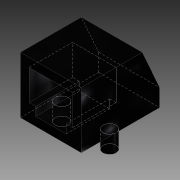
# Autodesk Inventor part: 6P6C
Saved by Autodesk Inventor 2014 (Build 180170000, 170)
## iProperties
Created: 2014-04-06
Part Number: 6P6C
Material: PC/ABS Plastic
Document SubType Name: Modeling
Designer: Tyler
Density: 0.357273 g/cm^3
Appearance: Smooth - White
Author: Tyler
Autodesk Inventor part; units mm, degrees
ref_plane "YZ Plane" through (0, 0, 0) normal (1, 0, 0) x (0, 1, 0)
ref_plane "XZ Plane" through (0, 0, 0) normal (0, 1, 0) x (-1, 0, 0)
ref_plane "XY Plane" through (0, 0, 0) normal (0, 0, 1) x (1, 0, 0)
sketch "Sketch1" plane through (0, 0, 0) normal (1, 0, 0) x (0, 1, 0)
  line L0 (-9, 13) -> (-9, 0)
  line L1 (-9, 0) -> (9, 0)
  line L2 (9, 0) -> (9, 4)
  line L3 (9, 4) -> (5, 13)
  line L4 (5, 13) -> (-9, 13)
  point P0 (0, 0)
  dimension "d0" = 13
  dimension "d1" = 18
  dimension "d2" = 9
  dimension "d3" = 0
  dimension "d4" = 4
  dimension "d5" = 14
  constraints: 10 end point, 2 parallel, 1 perpendicular, 1 vertical
  measures "d0" distance of L0.start L0.end
  measures "d1" distance of L0.end L1.end
  measures "d2" distance from line of point (0, 0) L0
  measures "d3" distance from line of L1 point (0, 0)
  measures "d4" distance of L1.end L2.end
  measures "d5" distance of L3.end L0.start
extrude "Extrusion1" add sketch "Sketch1" along normal blind 14
sketch "Sketch2" plane through (0, -9, 0) normal (0, -1, 0) x (1, 0, 0)
  line L0 (0, 13) -> (0, 0) projected
  line L1 (14, 13) -> (14, 0) projected
  line L2 (0, 13) -> (14, 13) projected
  line L3 (2, 11) -> (12, 11)
  line L4 (12, 11) -> (12, 4)
  line L5 (12, 4) -> (2, 4)
  line L6 (2, 4) -> (2, 11)
  line L7 (3.5, 2) -> (10.5, 2)
  line L8 (10.5, 2) -> (10.5, 4)
  line L9 (10.5, 4) -> (3.5, 4)
  line L10 (3.5, 4) -> (3.5, 2)
  dimension "d8" = 10
  dimension "d9" = 7
  dimension "d10" = 2
  dimension "d11" = 2
  dimension "d12" = 2
  dimension "d13" = 7
  dimension "d14" = 2
  dimension "d15" = 0
  dimension "d16" = 3.5
  constraints: 16 end point, 4 parallel, 2 horizontal, 2 perpendicular
  measures "d8" distance between parallel lines of L4 L6
  measures "d9" distance between parallel lines of L5 L3
  measures "d10" distance between parallel lines of L2 L3
  measures "d11" distance between parallel lines of L4 L1
  measures "d12" distance between parallel lines of L0 L6
  measures "d13" distance of L8.end L9.end
  measures "d14" distance of L9.end L7.start
  measures "d15" distance between parallel lines of L5 L9
  measures "d16" distance between parallel lines of L0 L10
extrude "Extrusion2" cut sketch "Sketch2" against normal blind 10
sketch "Sketch3" plane through (0, -9, 0) normal (0, 0, -1) x (-1, 0, 0)
  line L0 (0, 0) -> (0, 18) projected
  line L1 (-14, 0) -> (-14, 18) projected
  line L2 (0, 0) -> (-14, 0) projected
  circle A0 centre (-12.5, 8) radius 1.5
  circle A1 centre (-1.5, 8) radius 1.5
  point P0 (0, 9)
  dimension "d19" = 3
  dimension "d20" = 1.5
  dimension "d21" = 1.5
  dimension "d22" = 8
  dimension "d23" = 8
  constraints: 2 centre point, 1 equal radius
  measures "d19" diameter of A1
  measures "d20" distance from line of L0 A1.centre
  measures "d21" distance from line of L1 A0.centre
  measures "d22" distance from line of L2 A0.centre
  measures "d23" distance from line of L2 A1.centre
extrude "Extrusion3" add sketch "Sketch3" along normal blind 4
equation "\"d2\" = 0.5 * d1"
equation "\"d11\" = d12"
body "Solid1"
